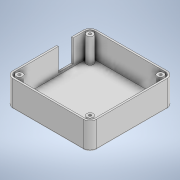
# Autodesk Inventor part: Arduino_case_bottom_JC_Rev1
Saved by Autodesk Inventor 2020 (Build 240168000, 168)
## iProperties
Created: 2019-08-28
Part Number: Arduino_case_bottom_JC_Rev1
Material: Generic
Document SubType Name: Modeling
Designer: jcocker
Density: 1 g/cm^3
Appearance: Default
Author: jcocker
Autodesk Inventor part; units mm, degrees
ref_plane "YZ Plane" through (0, 0, 0) normal (1, 0, 0) x (0, 1, 0)
ref_plane "XZ Plane" through (0, 0, 0) normal (0, 1, 0) x (-1, 0, 0)
ref_plane "XY Plane" through (0, 0, 0) normal (0, 0, 1) x (1, 0, 0)
sketch "Sketch1" plane through (0, 0, 0) normal (0, 1, 0) x (-1, 0, 0)
  line L0 (-33.65, -40) -> (33.65, -40)
  line L1 (40, -33.65) -> (40, 33.65)
  line L2 (33.65, 40) -> (-33.65, 40)
  line L3 (-40, 33.65) -> (-40, -33.65)
  line L4 (-40, -40) -> (40, 40) construction
  line L5 (40, -40) -> (-40, 40) construction
  arc A0 (40, 33.65) -> (33.65, 40) centre (33.65, 33.65) ccw
  arc A1 (-33.65, 40) -> (-40, 33.65) centre (-33.65, 33.65) ccw
  arc A2 (-40, -33.65) -> (-33.65, -40) centre (-33.65, -33.65) ccw
  arc A3 (33.65, -40) -> (40, -33.65) centre (33.65, -33.65) ccw
  point P0 (0, 0)
  dimension "d0" = 80
  dimension "d1" = 80
  dimension "d2" = 6.35
  constraints: 12 end point, 8 point on circle, 8 point on line, 8 tangent, 4 centre point, 3 equal radius, 2 midpoint, 2 parallel, 1 horizontal, 1 perpendicular
  measures "d0" distance of L5.end L4.end
  measures "d1" distance of L4.end L5.start
  measures "d2" radius of A0
extrude "Extrusion1" add sketch "Sketch1" along normal blind 25.4
shell "Shell1" thickness 1.7 removed faces 1 at (-11.2167, 25.4, 9.1)
fillet "Fillet1" radius 1.27 8 edges at (-38.1401, 0, -38.1401) (-40, 0, 0) (-38.1401, 0, 38.1401) (0, 0, 40) (38.1401, 0, 38.1401) (40, 0, 0) (38.1401, 0, -38.1401) (0, 0, -40)
sketch "Sketch2" plane through (-33.65, 1.7, 38.3) normal (0, 1, 0) x (1, 0, 0)
  arc A0 (-4.65, 4.65) -> (0, 0) centre (0, 4.65) ccw projected
  circle A1 centre (0, 4.65) radius 3.175
  circle A2 centre (0, 4.65) radius 1.2
  point P0 (33.65, 38.3)
  dimension "d7" = 6.35
  dimension "d8" = 2.4
  constraints: 2 centre point, 2 coincident
  measures "d7" diameter of A1
  measures "d8" diameter of A2
extrude "Extrusion2" add sketch "Sketch2" along normal up to surface (23.7 mm away)
mirror "Mirror1" about plane through (0, 0, 0) normal (1, 0, 0) of "Extrusion2"
mirror "Mirror2" about plane through (0, 0, 0) normal (0, 0, 1) of "Extrusion2", "Mirror1"
sketch "Sketch3" plane through (-40, 25.4, -33.65) normal (-1, 0, 0) x (0, 0, 1)
  line L0 (0, 0) -> (67.3, 0) projected
  line L1 (11.43, 0) -> (25.43, 0)
  line L2 (25.43, 0) -> (25.43, -21.59)
  line L3 (25.43, -21.59) -> (11.43, -21.59)
  line L4 (11.43, -21.59) -> (11.43, 0)
  line L5 (-6.35, -24.13) -> (-6.35, 0) projected
  point P0 (33.65, -25.4)
  dimension "d11" = 14
  dimension "d12" = 21.59
  dimension "d13" = 17.78
  constraints: 8 end point, 2 parallel, 1 horizontal, 1 perpendicular, 1 point on line
  measures "d11" distance of L2.end L3.end
  measures "d12" distance of L1.end L2.end
  measures "d13" distance between parallel lines of L5 L4
extrude "Extrusion3" cut sketch "Sketch3" against normal blind 25.4
body "Solid1"
